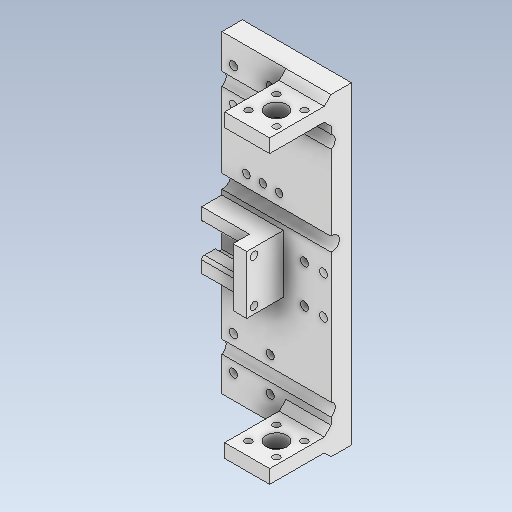
# Autodesk Inventor part: 0008-10-008 X Axis suport
Saved by Autodesk Inventor 2020 (Build 240168000, 168)
## iProperties
Created: 2021-02-27
Part Number: 0008-10-008 X Axis suport
Material: ABS Plastic
Document SubType Name: Modeling
Designer: Iulian Bors
Density: 1.06 g/cm^3
Appearance: Smooth - White
Mass: 328.084 g
Surface Area: 644.049 cm^2
Volume: 309.513 cm^3
Description: Suport Axa X
Author: Iulian Bors
Subject: 008
Autodesk Inventor part; units mm, degrees
ref_plane "YZ Plane" through (0, 0, 0) normal (1, 0, 0) x (0, 1, 0)
ref_plane "XZ Plane" through (0, 0, 0) normal (0, 1, 0) x (-1, 0, 0)
ref_plane "XY Plane" through (0, 0, 0) normal (0, 0, 1) x (1, 0, 0)
sketch "Sketch1" plane through (0, 0, 0) normal (0, 0, 1) x (1, 0, 0)
  line L0 (-40, 115) -> (40, 115)
  line L1 (40, 115) -> (40, -115)
  line L2 (40, -115) -> (-40, -115)
  line L3 (-40, -115) -> (-40, 115)
  point P0 (0, 0)
  point P1 (0, 115)
  point P2 (-40, 0)
  dimension "d0" = 230
  dimension "d1" = 80
  constraints: 8 end point, 2 midpoint, 2 parallel, 1 horizontal, 1 horizontal alignment, 1 perpendicular, 1 vertical alignment
  measures "d0" distance of L2.end L0.start
  measures "d1" distance of L1.end L2.end
extrude "Extrusion1" add sketch "Sketch1" along normal blind 15
sketch "Sketch2" plane through (40, -115, 0) normal (1, 0, 0) x (0, 0, -1)
  circle A0 centre (-17, 30) radius 5.15
  circle A1 centre (-17, 200) radius 5.15
  line L0 (-15, 0) -> (-15, 230) projected
  line L1 (0, 230) -> (-15, 230) projected
  line L2 (0, 0) -> (-15, 0) projected
  point P0 (0, 115)
  dimension "d4" = 10.3
  dimension "d5" = 2
  dimension "d6" = 30
  dimension "d7" = 2
  dimension "d8" = 30
  constraints: 2 centre point, 1 equal radius
  measures "d4" diameter of A1
  measures "d5" distance from line of L0 A1.centre
  measures "d6" distance from line of L1 A1.centre
  measures "d7" distance from line of A0.centre L0
  measures "d8" distance from line of A0.centre L2
extrude "Extrusion2" cut sketch "Sketch2" against normal through all
sketch "Sketch3" plane through (-40, -115, 0) normal (-1, 0, 0) x (0, 0, 1)
  circle A0 centre (14, 135) radius 5.15
  line L0 (15, 195.2542) -> (15, 34.7458) projected
  line L1 (0, 0) -> (15, 0) projected
  point P0 (0, 115)
  dimension "d11" = 1
  dimension "d12" = 10.3
  dimension "d13" = 135
  constraints: 1 centre point
  measures "d11" distance from line of L0 A0.centre
  measures "d12" diameter of A0
  measures "d13" distance from line of A0.centre L1
extrude "Extrusion3" cut sketch "Sketch3" against normal through all
sketch "Sketch5" plane through (-40, -115, 0) normal (-1, 0, 0) x (0, 0, 1)
  line L0 (19.8, 118.25) -> (19.8, 115.55)
  line L1 (15, 118.25) -> (19.8, 118.25)
  line L2 (15, 91.75) -> (15, 118.25)
  line L3 (15, 91.75) -> (19.8, 91.75)
  line L4 (19.8, 94.45) -> (19.8, 91.75)
  line L5 (26.9188, 105) -> (15, 105) construction
  line L6 (15, 129.948) -> (15, 34.7458) construction
  line L7 (0, 0) -> (15, 0) construction
  line L8 (0, 0) -> (15, 0) construction
  line L9 (19.8, 115.55) -> (29.8, 115.55)
  line L10 (29.8, 115.55) -> (29.8, 126.25)
  line L11 (29.8, 126.25) -> (15, 126.25)
  line L12 (15, 126.25) -> (15, 118.25)
  line L13 (19.8, 94.45) -> (29.8, 94.45)
  line L14 (29.8, 94.45) -> (29.8, 83.75)
  line L15 (29.8, 83.75) -> (15, 83.75)
  line L16 (15, 83.75) -> (15, 91.75)
  point P0 (0, 115)
  dimension "d20" = 26.5
  dimension "d21" = 4.8
  dimension "d26" = 13.25
  dimension "d28" = 105
  dimension "d29" = 2.7
  dimension "d30" = 10
  dimension "d31" = 8
  constraints: 28 end point, 6 perpendicular, 3 symmetric about line, 2 collinear, 2 equal length, 2 point on line, 1 horizontal
  measures "d20" distance of L2.start L1.start
  measures "d21" distance of L1.start L0.start
  measures "d26" distance between parallel lines of L3 L5
  measures "d28" distance between parallel lines of L8 L5
  measures "d29" distance of L0.start L0.end
  measures "d30" distance of L0.end L9.end
  measures "d31" distance between parallel lines of L1 L11
extrude "Extrusion4" add sketch "Sketch5" against normal blind 35
fillet "Fillet1" radius 2 2 edges at (-22.5, 0.55, 29.8) (-22.5, -20.55, 29.8)
sketch "Sketch6" plane through (-5, -115, 0) normal (1, 0, 0) x (0, 0, -1)
  line L0 (-29.8, 83.75) -> (-15, 83.75) projected
  line L1 (-15, 83.75) -> (-41.8, 83.75)
  line L2 (-41.8, 83.75) -> (-41.8, 126.25)
  line L3 (-41.8, 126.25) -> (-15, 126.25)
  line L4 (-15, 126.25) -> (-15, 83.75)
  line L5 (-15, 126.25) -> (-29.8, 126.25) projected
  line L6 (-29.8, 92.45) -> (-29.8, 83.75) projected
  point P0 (0, 115)
  dimension "d35" = 12
  constraints: 8 end point, 2 parallel, 1 collinear, 1 horizontal, 1 perpendicular
  measures "d35" distance between parallel lines of L6 L2
extrude "Extrusion5" add sketch "Sketch6" along normal blind 10
sketch "Sketch7" plane through (-5, -115, 0) normal (-1, 0, 0) x (0, 0, 1)
  circle A0 centre (36.5, 121) radius 2.25 projected
  circle A1 centre (36.5, 89) radius 2.25 projected
  point P0 (0, 115)
hole "Hole1" at (-5, 6, 36.5) at (-5, -26, 36.5) direction (1, 0, 0) diameter 5.5 end through all
sketch "Sketch8" plane through (0, 0, 15) normal (0, 0, 1) x (1, 0, 0)
  line L0 (40, -110) -> (7, -110)
  line L1 (7, -110) -> (7, -100)
  line L2 (7, -100) -> (40, -100)
  line L3 (40, -100) -> (40, -110)
  line L4 (-40, -115) -> (40, -115)
  line L5 (40, -115) -> (40, -89.7458)
  line L6 (40, -115) -> (40, -89.7458) projected
  point P0 (0, 0)
  point P1 (0, 0)
  dimension "d47" = 33
  dimension "d48" = 5
  dimension "d49" = 10
  constraints: 12 end point, 2 collinear, 2 parallel, 1 horizontal, 1 perpendicular
  measures "d47" distance of L0.start L0.end
  measures "d48" distance between parallel lines of L4 L0
  measures "d49" distance between parallel lines of L0 L2
extrude "Extrusion6" add sketch "Sketch8" along normal blind 45
sketch "Sketch9" plane through (7, -100, 15) normal (0, 1, 0) x (1, 0, 0)
  circle A0 centre (28.253, -35.253) radius 2.5
  circle A1 centre (7.747, -35.253) radius 2.5
  circle A2 centre (7.747, -14.747) radius 2.5
  circle A3 centre (18, -25) radius 7.5
  circle A4 centre (28.253, -14.747) radius 2.5
  line L0 (0, 0) -> (33, 0) projected
  line L1 (33, 0) -> (33, -45) projected
  line L2 (33, -45) -> (0, -45) projected
  line L3 (0, 0) -> (0, -45) projected
  point P0 (-7, 15)
  dimension "d55" = 20.5061
  dimension "d59" = 15
  dimension "d61" = 20.5061
  dimension "d62" = 5
  dimension "d63" = 4.747
  dimension "d65" = 20
  dimension "d66" = 18
  dimension "d95" = 10.253
  constraints: 5 centre point, 3 equal radius, 2 horizontal alignment, 2 vertical alignment
  measures "d55" distance of A1.centre A0.centre
  measures "d59" diameter of A3
  measures "d61" distance of A0.centre A4.centre
  measures "d62" diameter of A0
  measures "d63" distance from line of L1 A4.centre
  measures "d65" distance from line of L2 A3.centre
  measures "d66" distance from line of L3 A3.centre
  measures "d95" horizontal distance of A3.centre A4.centre
extrude "Extrusion7" cut sketch "Sketch9" against normal through all contours A0 | A1 | A2 | A3 | A4
sketch "Sketch10" plane through (7, -110, 60) normal (0, -1, 0) x (1, 0, 0)
  circle A0 centre (28.253, -30.253) radius 2.5 projected
  line L0 (33, -45) -> (33, 0) projected
  line L1 (0, 0) -> (33, 0) projected
  line L2 (0, -45) -> (0, 0) projected
  circle A1 centre (7.747, -30.253) radius 2.5 projected
  circle A2 centre (18, -20) radius 7.5 projected
  circle A3 centre (7.747, -9.747) radius 2.5 projected
  circle A4 centre (28.253, -9.747) radius 2.5 projected
  circle A5 centre (7.747, -30.253) radius 4.5
  circle A6 centre (28.253, -30.253) radius 4.5
  line L3 (33, -45) -> (0, -45) projected
  point P0 (-7, -60)
  dimension "d78" = 9
  constraints: 2 centre point, 2 coincident, 1 equal radius
  measures "d78" diameter of A5
extrude "Extrusion8" cut sketch "Sketch10" along normal blind 35 contours A0 | A1 | A5 | A6
mirror "Mirror2" about plane through (0, 0, 0) normal (0, 1, 0) of "Extrusion8", "Extrusion7", "Extrusion6"
sketch "Sketch11" plane through (0, 0, 0) normal (0, 0, -1) x (-1, 0, 0)
  circle A0 centre (-20.5, -1) radius 2.5
  circle A1 centre (-34.5, -1) radius 2.5
  circle A2 centre (-20.5, -29) radius 2.5
  circle A3 centre (-34.5, -29) radius 2.5
  line L0 (-34.5, -1) -> (-20.5, -1) construction
  line L1 (-20.5, -1) -> (-20.5, -29) construction
  line L2 (-20.5, -29) -> (-34.5, -29) construction
  line L3 (-34.5, -29) -> (-34.5, -1) construction
  line L4 (-40, -115) -> (-40, 115) projected
  line L5 (40, -115) -> (-40, -115) projected
  circle A4 centre (31.5, 72.425) radius 2.75 projected
  circle A5 centre (31.5, 97.575) radius 2.75 projected
  circle A6 centre (4.5, 97.575) radius 2.75 projected
  circle A7 centre (4.5, 72.425) radius 2.75 projected
  circle A8 centre (4.5, -72.425) radius 2.75 projected
  circle A9 centre (4.5, -97.575) radius 2.75 projected
  circle A10 centre (31.5, -97.575) radius 2.75 projected
  circle A11 centre (31.5, -72.425) radius 2.75 projected
  point P0 (0, 0)
  dimension "d82" = 5.5
  dimension "d84" = 86
  dimension "d85" = 14
  dimension "d86" = 28
  dimension "d87" = 5
  constraints: 8 end point, 4 centre point, 3 coincident, 3 equal radius, 2 parallel, 1 horizontal, 1 perpendicular
  measures "d82" distance between parallel lines of L4 L3
  measures "d84" distance between parallel lines of L5 L2
  measures "d85" distance of A0.centre L0.start
  measures "d86" distance of L2.end L0.start
  measures "d87" diameter of A1
hole "Hole2" at (20.5, -1, 0) at (34.5, -1, 0) at (34.5, -29, 0) at (20.5, -29, 0) at (-4.5, 97.575, 0) at (-31.5, 97.575, 0) at (-31.5, 72.425, 0) at (-4.5, 72.425, 0) at (-31.5, -72.425, 0) at (-31.5, -97.575, 0) at (-4.5, -97.575, 0) at (-4.5, -72.425, 0) direction (0, 0, 1) diameter 6 end through all
chamfer "Chamfer4" distance 5 angle 45 4 edges at (23.5, -100, 15) (23.5, -110, 15) (23.5, 110, 15) (23.5, 100, 15)
sketch "Sketch13" plane through (0, 0, 15) normal (0, 0, 1) x (1, 0, 0)
  circle A0 centre (-22, 33.593) radius 2.75 projected
  circle A1 centre (-10, 33.593) radius 2.75 projected
  circle A2 centre (2, 33.593) radius 2.75 projected
  point P0 (0, 0)
extrude "Extrusion10" cut sketch "Sketch13" against normal through all
equation "\"d7\" = d5"
equation "\"d8\" = d6"
equation "\"d26\" = 0.5 * d20"
body "Solid1"
